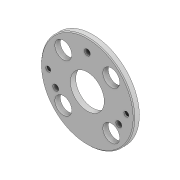
# Autodesk Inventor part: AMT102Mount
Saved by Autodesk Inventor 2021 (Build 250183000, 183)
## iProperties
Created: 2020-08-06
Part Number: AMT102Mount
Material: Generic
Document SubType Name: Modeling
Designer: Derm
Density: 1 g/cm^3
Appearance: Default
Author: Derm
Autodesk Inventor part; units mm, degrees
ref_plane "YZ Plane" through (0, 0, 0) normal (1, 0, 0) x (0, 1, 0)
ref_plane "XZ Plane" through (0, 0, 0) normal (0, 1, 0) x (-1, 0, 0)
ref_plane "XY Plane" through (0, 0, 0) normal (0, 0, 1) x (1, 0, 0)
sketch "Sketch1" plane through (0, 0, 0) normal (0, 0, 1) x (1, 0, 0)
  circle A0 centre (-43.950789, -25.375) radius 1.8
  circle A1 centre (0, -50.75) radius 1.8
  circle A2 centre (43.950789, -25.375) radius 1.8
  circle A3 centre (43.950789, 25.375) radius 1.8
  circle A4 centre (0, 50.75) radius 1.8
  circle A5 centre (-43.950789, 25.375) radius 1.8
  circle A6 centre (0, 0) radius 55
  circle A7 centre (0, 0) radius 10
  line L0 (-5, -45.365185) -> (-5, -28.788018)
  arc A8 (-3.318966, -27.298983) -> (-5, -28.788018) centre (-3.5, -28.788018) ccw
  arc A9 (-3.318966, -27.298983) -> (3.318966, -27.298983) centre (0, 0) ccw
  arc A10 (5, -28.788018) -> (3.318966, -27.298983) centre (3.5, -28.788018) ccw
  line L1 (5, -28.788018) -> (5, -45.365185)
  arc A11 (3.615385, -46.86074) -> (5, -45.365185) centre (3.5, -45.365185) ccw
  arc A12 (-3.615385, -46.86074) -> (3.615385, -46.86074) centre (0, 0) ccw
  arc A13 (-5, -45.365185) -> (-3.615385, -46.86074) centre (-3.5, -45.365185) ccw
  arc A14 (3.615385, 46.86074) -> (-3.615385, 46.86074) centre (0, 0) ccw
  arc A15 (5, 45.365185) -> (3.615385, 46.86074) centre (3.5, 45.365185) ccw
  line L2 (5, 45.365185) -> (5, 28.788018)
  arc A16 (3.318966, 27.298983) -> (5, 28.788018) centre (3.5, 28.788018) ccw
  arc A17 (3.318966, 27.298983) -> (-3.318966, 27.298983) centre (0, 0) ccw
  arc A18 (-5, 28.788018) -> (-3.318966, 27.298983) centre (-3.5, 28.788018) ccw
  line L3 (-5, 28.788018) -> (-5, 45.365185)
  arc A19 (-3.615385, 46.86074) -> (-5, 45.365185) centre (-3.5, 45.365185) ccw
  circle A20 centre (25.375, -43.950789) radius 3.75
  arc A21 (11.879121, -45.47402) -> (23.5, -40.703194) centre (0, 0) ccw
  arc A22 (10, -44.022721) -> (11.879121, -45.47402) centre (11.5, -44.022721) ccw
  line L4 (10, -44.022721) -> (10, -26.622359)
  arc A23 (10.905172, -25.24534) -> (10, -26.622359) centre (11.5, -26.622359) ccw
  arc A24 (10.905172, -25.24534) -> (25.24534, -10.905172) centre (0, 0) ccw
  arc A25 (26.622359, -10) -> (25.24534, -10.905172) centre (26.622359, -11.5) ccw
  line L5 (26.622359, -10) -> (44.022721, -10)
  arc A26 (45.47402, -11.879121) -> (44.022721, -10) centre (44.022721, -11.5) ccw
  arc A27 (23.5, -40.703194) -> (45.47402, -11.879121) centre (0, 0) ccw
  circle A28 centre (-50.75, 0) radius 3.75
  arc A29 (-46.86074, 3.615385) -> (-47, 0) centre (0, 0) ccw
  arc A30 (-45.365185, 5) -> (-46.86074, 3.615385) centre (-45.365185, 3.5) ccw
  line L6 (-45.365185, 5) -> (-28.788018, 5)
  arc A31 (-27.298983, 3.318966) -> (-28.788018, 5) centre (-28.788018, 3.5) ccw
  arc A32 (-27.298983, 3.318966) -> (-27.298983, -3.318966) centre (0, 0) ccw
  arc A33 (-28.788018, -5) -> (-27.298983, -3.318966) centre (-28.788018, -3.5) ccw
  line L7 (-28.788018, -5) -> (-45.365185, -5)
  arc A34 (-46.86074, -3.615385) -> (-45.365185, -5) centre (-45.365185, -3.5) ccw
  arc A35 (-47, 0) -> (-46.86074, -3.615385) centre (0, 0) ccw
  circle A36 centre (25.375, 43.950789) radius 3.75
  arc A37 (45.47402, 11.879121) -> (23.5, 40.703194) centre (0, 0) ccw
  arc A38 (44.022721, 10) -> (45.47402, 11.879121) centre (44.022721, 11.5) ccw
  line L8 (44.022721, 10) -> (26.622359, 10)
  arc A39 (25.24534, 10.905172) -> (26.622359, 10) centre (26.622359, 11.5) ccw
  arc A40 (25.24534, 10.905172) -> (10.905172, 25.24534) centre (0, 0) ccw
  arc A41 (10, 26.622359) -> (10.905172, 25.24534) centre (11.5, 26.622359) ccw
  line L9 (10, 26.622359) -> (10, 44.022721)
  arc A42 (11.879121, 45.47402) -> (10, 44.022721) centre (11.5, 44.022721) ccw
  arc A43 (23.5, 40.703194) -> (11.879121, 45.47402) centre (0, 0) ccw
  circle A44 centre (-25.375, 43.950789) radius 3.75
  arc A45 (-11.879121, 45.47402) -> (-23.5, 40.703194) centre (0, 0) ccw
  arc A46 (-10, 44.022721) -> (-11.879121, 45.47402) centre (-11.5, 44.022721) ccw
  line L10 (-10, 44.022721) -> (-10, 26.622359)
  arc A47 (-10.905172, 25.24534) -> (-10, 26.622359) centre (-11.5, 26.622359) ccw
  arc A48 (-10.905172, 25.24534) -> (-25.24534, 10.905172) centre (0, 0) ccw
  arc A49 (-26.622359, 10) -> (-25.24534, 10.905172) centre (-26.622359, 11.5) ccw
  line L11 (-26.622359, 10) -> (-44.022721, 10)
  arc A50 (-45.47402, 11.879121) -> (-44.022721, 10) centre (-44.022721, 11.5) ccw
  arc A51 (-23.5, 40.703194) -> (-45.47402, 11.879121) centre (0, 0) ccw
  circle A52 centre (-25.375, -43.950789) radius 3.75
  arc A53 (-45.47402, -11.879121) -> (-23.5, -40.703194) centre (0, 0) ccw
  arc A54 (-44.022721, -10) -> (-45.47402, -11.879121) centre (-44.022721, -11.5) ccw
  line L12 (-44.022721, -10) -> (-26.622359, -10)
  arc A55 (-25.24534, -10.905172) -> (-26.622359, -10) centre (-26.622359, -11.5) ccw
  arc A56 (-25.24534, -10.905172) -> (-10.905172, -25.24534) centre (0, 0) ccw
  arc A57 (-10, -26.622359) -> (-10.905172, -25.24534) centre (-11.5, -26.622359) ccw
  line L13 (-10, -26.622359) -> (-10, -44.022721)
  arc A58 (-11.879121, -45.47402) -> (-10, -44.022721) centre (-11.5, -44.022721) ccw
  arc A59 (-23.5, -40.703194) -> (-11.879121, -45.47402) centre (0, 0) ccw
  circle A60 centre (50.75, 0) radius 3.75
  arc A61 (46.86074, -3.615385) -> (47, 0) centre (0, 0) ccw
  arc A62 (45.365185, -5) -> (46.86074, -3.615385) centre (45.365185, -3.5) ccw
  line L14 (45.365185, -5) -> (28.788018, -5)
  arc A63 (27.298983, -3.318966) -> (28.788018, -5) centre (28.788018, -3.5) ccw
  arc A64 (27.298983, -3.318966) -> (27.298983, 3.318966) centre (0, 0) ccw
  arc A65 (28.788018, 5) -> (27.298983, 3.318966) centre (28.788018, 3.5) ccw
  line L15 (28.788018, 5) -> (45.365185, 5)
  arc A66 (46.86074, 3.615385) -> (45.365185, 5) centre (45.365185, 3.5) ccw
  arc A67 (47, 0) -> (46.86074, 3.615385) centre (0, 0) ccw
  circle A68 centre (-14.142136, -14.142136) radius 5
  circle A69 centre (14.142136, 14.142136) radius 5
  circle A70 centre (-14.142136, 14.142136) radius 5
  circle A71 centre (14.142136, -14.142136) radius 5
  circle A72 centre (0, 0) radius 27.5
  circle A73 centre (0, 20) radius 1.75
  circle A74 centre (-18.600039, -7.351092) radius 1.75
  circle A75 centre (18.59999, -7.351217) radius 1.75
  point P0 (0, 0)
  point P1 (-27.298983, -3.318966)
  point P2 (-25.24534, -10.905172)
  point P3 (-10.905172, -25.24534)
  point P4 (3.318966, -27.298983)
  point P5 (25.24534, -10.905172)
  point P6 (27.298983, 3.318966)
  point P7 (25.24534, 10.905172)
  point P8 (10.905172, 25.24534)
  point P9 (-3.318966, 27.298983)
  point P10 (-25.24534, 10.905172)
  constraints: 2 horizontal alignment, 1 centre point, 1 coincident, 4 other
sketch "Sketch1 outline for Extrusion1" plane through (0, 0, 0) normal (0, 0, 1) x (1, 0, 0)
  arc A0 (-27.298983, -3.318966) -> (-25.24534, -10.905172) centre (0, 0) ccw
  arc A1 (-27.298983, 3.318966) -> (-27.298983, -3.318966) centre (0, 0) ccw
  arc A2 (-25.24534, -10.905172) -> (-10.905172, -25.24534) centre (0, 0) ccw
  arc A3 (-25.24534, 10.905172) -> (-27.298983, 3.318966) centre (0, 0) ccw
  arc A4 (-10.905172, -25.24534) -> (-3.318966, -27.298983) centre (0, 0) ccw
  arc A5 (-10.905172, 25.24534) -> (-25.24534, 10.905172) centre (0, 0) ccw
  arc A6 (-3.318966, -27.298983) -> (3.318966, -27.298983) centre (0, 0) ccw
  arc A7 (-3.318966, 27.298983) -> (-10.905172, 25.24534) centre (0, 0) ccw
  arc A8 (3.318966, -27.298983) -> (10.905172, -25.24534) centre (0, 0) ccw
  arc A9 (3.318966, 27.298983) -> (-3.318966, 27.298983) centre (0, 0) ccw
  arc A10 (10.905172, -25.24534) -> (25.24534, -10.905172) centre (0, 0) ccw
  arc A11 (10.905172, 25.24534) -> (3.318966, 27.298983) centre (0, 0) ccw
  arc A12 (25.24534, -10.905172) -> (27.298983, -3.318966) centre (0, 0) ccw
  arc A13 (25.24534, 10.905172) -> (10.905172, 25.24534) centre (0, 0) ccw
  arc A14 (27.298983, -3.318966) -> (27.298983, 3.318966) centre (0, 0) ccw
  arc A15 (27.298983, 3.318966) -> (25.24534, 10.905172) centre (0, 0) ccw
  circle A16 centre (-14.142136, -14.142136) radius 5
  circle A17 centre (-18.600039, -7.351092) radius 1.75
  circle A18 centre (14.142136, -14.142136) radius 5
  circle A19 centre (0, 0) radius 10
  circle A20 centre (18.59999, -7.351217) radius 1.75
  circle A21 centre (-14.142136, 14.142136) radius 5
  circle A22 centre (0, 20) radius 1.75
  circle A23 centre (14.142136, 14.142136) radius 5
extrude "Extrusion1" add sketch "Sketch1 outline for Extrusion1" along normal blind 3.175
sketch "Sketch2" plane through (0, 0, 3.175) normal (0, 0, 1) x (1, 0, 0)
  circle A0 centre (-23.0125, 0) radius 1.435 projected
  circle A1 centre (23.0125, 0) radius 1.435 projected
  point P0 (0, 0)
extrude "Extrusion2" cut sketch "Sketch2" against normal blind 3.175
sketch "Sketch3" plane through (0, 0, 0) normal (0, 0, -1) x (-1, 0, 0)
  circle A0 centre (-23.0125, 0) radius 1.435
  circle A1 centre (23.0125, 0) radius 1.435
  line L0 (-23.0125, 3.175426) -> (-20.2625, 1.587713)
  line L1 (-20.2625, 1.587713) -> (-20.2625, -1.587713)
  line L2 (-20.2625, -1.587713) -> (-23.0125, -3.175426)
  line L3 (-23.0125, -3.175426) -> (-25.7625, -1.587713)
  line L4 (-25.7625, -1.587713) -> (-25.7625, 1.587713)
  line L5 (-25.7625, 1.587713) -> (-23.0125, 3.175426)
  circle A2 centre (23.0125, 0) radius 1.435
  line L6 (23.0125, 3.175426) -> (25.7625, 1.587713)
  line L7 (25.7625, 1.587713) -> (25.7625, -1.587713)
  line L8 (25.7625, -1.587713) -> (23.0125, -3.175426)
  line L9 (23.0125, -3.175426) -> (20.2625, -1.587713)
  line L10 (20.2625, -1.587713) -> (20.2625, 1.587713)
  line L11 (20.2625, 1.587713) -> (23.0125, 3.175426)
  point P0 (0, 0)
  dimension "d4" = 5.5
  dimension "d5" = 5.5
  constraints: 24 end point, 2 coincident, 26 other
  measures "d4" distance between parallel lines of L1 L4
  measures "d5" distance between parallel lines of L7 L10
extrude "Extrusion3" cut sketch "Sketch3" against normal blind 2.4
chamfer "Chamfer1" distance 0.5 angle 45 1 edges at (-25.2453, -10.9052, 3.175)
body "Solid1"
